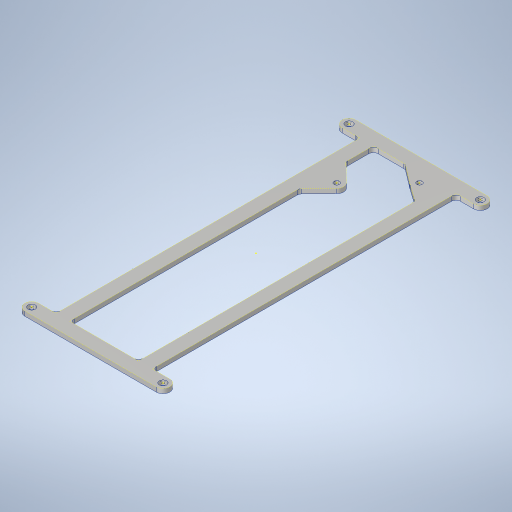
# Autodesk Inventor part: DB1-007
Saved by Autodesk Inventor 2023.4 (Build 274418000, 418)
## iProperties
Created: 2025-01-15
Part Number: DB1-007
Material: Aluminum 6061
Document SubType Name: Modeling
Designer: mavericks
Density: 2.7 g/cm^3
Appearance: Aluminum - Flat
Author: mavericks
Autodesk Inventor part; units mm, degrees
ref_plane "YZ Plane" through (0, 0, 0) normal (1, 0, 0) x (0, 1, 0)
ref_plane "XZ Plane" through (0, 0, 0) normal (0, 1, 0) x (-1, 0, 0)
ref_plane "XY Plane" through (0, 0, 0) normal (0, 0, 1) x (1, 0, 0)
sketch "Sketch1" plane through (0, 0, 0) normal (0, 1, 0) x (-1, 0, 0)
  line L0 (45.974, 111.125) -> (-45.974, 111.125) construction
  line L1 (45.974, 115.8875) -> (-45.974, 115.8875)
  line L2 (-45.974, 106.3625) -> (45.974, 106.3625)
  arc A0 (45.974, 106.3625) -> (45.974, 115.8875) centre (45.974, 111.125) ccw
  arc A1 (-45.974, 115.8875) -> (-45.974, 106.3625) centre (-45.974, 111.125) ccw
  line L3 (0, 111.125) -> (0, -111.125) construction
  line L4 (45.974, -111.125) -> (-45.974, -111.125) construction
  line L5 (45.974, -115.8875) -> (-45.974, -115.8875)
  line L6 (-45.974, -106.3625) -> (45.974, -106.3625) construction
  arc A2 (45.974, -115.8875) -> (45.974, -106.3625) centre (45.974, -111.125) ccw
  arc A3 (-45.974, -106.3625) -> (-45.974, -115.8875) centre (-45.974, -111.125) ccw
  line L7 (24.13, 106.3625) -> (24.13, -106.3625)
  line L8 (-24.13, 106.3625) -> (-24.13, -106.3625) construction
  line L9 (24.13, 0) -> (-24.13, 0) construction
  line L10 (33.655, 106.3625) -> (33.655, -106.3625)
  line L11 (-33.655, 106.3625) -> (-33.655, -106.3625)
  line L12 (-14.478, -100.0125) -> (14.478, -71.0565) construction
  circle A4 centre (14.478, -71.0565) radius 4.7625 construction
  circle A5 centre (-14.478, -100.0125) radius 4.7625 construction
  line L13 (-11.6004, -96.2177) -> (1.7778, -106.3625) construction
  line L14 (-11.7289, -96.1236) -> (-24.13, -87.3572) construction
  line L15 (45.974, -106.3625) -> (33.655, -106.3625)
  line L16 (1.7778, -106.3625) -> (24.13, -106.3625)
  line L17 (-24.13, -87.3572) -> (-24.13, 106.3625)
  line L18 (1.7778, -106.3625) -> (-11.6004, -96.2177)
  line L19 (-24.13, -87.3572) -> (-11.7289, -96.1236)
  arc A6 (-11.6004, -96.2177) -> (-11.7289, -96.1236) centre (-14.478, -100.0125) ccw
  line L20 (11.0632, -67.7367) -> (24.13, -54.2961)
  line L21 (11.1582, -74.4713) -> (24.13, -87.0822)
  arc A7 (11.1582, -67.6417) -> (11.1582, -74.4713) centre (14.478, -71.0565) ccw
  line L22 (-33.655, -106.3625) -> (-45.974, -106.3625)
  point P0 (0, 0)
  point P1 (0, 0)
  point P2 (0, -111.125)
  point P3 (0, 0)
  point P4 (0, -85.5345)
  dimension "d0" = 9.525
  dimension "d1" = 91.948
  dimension "d2" = 222.25
  dimension "d4" = 9.525
  dimension "d5" = 48.26
  dimension "d6" = 9.525
  dimension "d7" = 9.525
  dimension "d8" = 28.956
  dimension "d9" = 28.956
  dimension "d10" = 6.35
  dimension "d11" = 9.525
  dimension "d12" = 9.525
  dimension "d13" = 25.9078
  dimension "d14" = 19.0053
  dimension "d15" = 32.7861
  constraints: 50 end point, 18 point on circle, 12 tangent, 9 point on line, 8 centre point, 7 coincident, 7 midpoint, 5 parallel, 4 collinear, 3 vertical alignment, 2 concentric, 2 horizontal, 2 perpendicular, 1 vertical
  measures "d0" diameter of A1
  measures "d1" distance of L0.end L0.start
  measures "d2" distance of L3.start L3.end
  measures "d4" distance of L5.end L6.start
  measures "d5" distance between parallel lines of L8 L7
  measures "d6" distance between parallel lines of L7 L10
  measures "d7" distance between parallel lines of L8 L11
  measures "d8" horizontal distance of L12.start L12.end
  measures "d9" horizontal distance of L12.start L12.end
  measures "d10" distance from line of L6 L12.start
  measures "d11" diameter of A4
  measures "d12" diameter of A5
  measures "d13" distance of L8.end L13.end
  measures "d14" distance of L8.end L14.end
  measures "d15" distance of L20.end L21.end
extrude "Extrusion1" add sketch "Sketch1" along normal blind 3.175 contours A0 L2 A1 L1 | L10 L15 A2 L5 A3 L22 L11 L2 L17 L19 A6 L18 L16 L7 | L7 L21 A7 L20
sketch "Sketch2" plane through (0, 3.175, 0) normal (0, 1, 0) x (1, 0, 0)
  line L0 (33.655, 106.3625) -> (45.974, 106.3625) construction
  arc A0 (45.974, 106.3625) -> (45.974, 115.8875) centre (45.974, 111.125) ccw construction
  line L1 (45.974, 115.8875) -> (-45.974, 115.8875) construction
  arc A1 (-45.974, 115.8875) -> (-45.974, 106.3625) centre (-45.974, 111.125) ccw construction
  line L2 (-45.974, 106.3625) -> (-33.655, 106.3625) construction
  line L3 (-33.655, 106.3625) -> (-33.655, -106.3625) construction
  line L4 (-33.655, -106.3625) -> (-45.974, -106.3625) construction
  arc A2 (-45.974, -106.3625) -> (-45.974, -115.8875) centre (-45.974, -111.125) ccw construction
  line L5 (-45.974, -115.8875) -> (45.974, -115.8875) construction
  arc A3 (45.974, -115.8875) -> (45.974, -106.3625) centre (45.974, -111.125) ccw construction
  line L6 (45.974, -106.3625) -> (33.655, -106.3625) construction
  line L7 (33.655, -106.3625) -> (33.655, 106.3625) construction
  line L8 (24.13, -106.3625) -> (-24.13, -106.3625) construction
  line L9 (-24.13, -106.3625) -> (-24.13, 54.2961) construction
  line L10 (-24.13, 54.2961) -> (-11.0632, 67.7367) construction
  arc A4 (-11.0632, 67.7367) -> (-11.1582, 74.4713) centre (-14.478, 71.0565) ccw construction
  line L11 (-11.1582, 74.4713) -> (-24.13, 87.0822) construction
  line L12 (-24.13, 87.0822) -> (-24.13, 106.3625) construction
  line L13 (-24.13, 106.3625) -> (-1.7778, 106.3625) construction
  line L14 (-1.7778, 106.3625) -> (11.6004, 96.2177) construction
  arc A5 (11.6004, 96.2177) -> (11.7289, 96.1236) centre (14.478, 100.0125) ccw construction
  line L15 (11.7289, 96.1236) -> (24.13, 87.3572) construction
  line L16 (24.13, 87.3572) -> (24.13, -106.3625) construction
  point P0 (0, 0)
  constraints: 6 coincident
hole "Hole1" at (-45.974, 3.175, 111.125) at (45.974, 3.175, 111.125) at (45.974, 3.175, -111.125) at (-45.974, 3.175, -111.125) direction (0, -1, 0) diameter 5.1054 end through all clearance for "Flat Head Machine Screw (82)" size "#10" standard "Ansi Unified Screw Threads"
hole "Hole2" at (-14.478, 3.175, -71.0565) at (14.478, 3.175, -100.0125) direction (0, -1, 0) diameter 3.81 end through all clearance for "Flat Head Machine Screw (82)" size "#6" standard "Ansi Unified Screw Threads"
fillet "Fillet1" radius 3.302 11 edges at (-24.13, 1.5875, -54.2961) (-24.13, 1.5875, -87.0822) (-24.13, 1.5875, -106.3625) (-1.7778, 1.5875, -106.3625) (24.13, 1.5875, -87.3572) (33.655, 1.5875, -106.3625) (-33.655, 1.5875, -106.3625) (-33.655, 1.5875, 106.3625) (-24.13, 1.5875, 106.3625) (24.13, 1.5875, 106.3625) (33.655, 1.5875, 106.3625)
equation "\"d4\" = d0"
equation "\"d6\" = d7"
body "Solid1"
